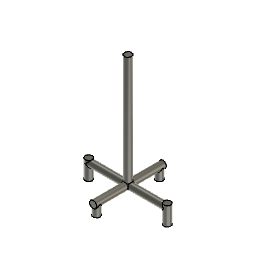
Quad-Ended Pendulum v1 (Autodesk Fusion 360 design; units mm, degrees)
Autodesk Fusion 360 part; units mm, degrees
sketch "Sketch1" plane through (0, 0, 0) normal (0, 0, 1) x (1, 0, 0)
  circle A0 centre (-42, 0) radius 8
  circle A1 centre (138, 0) radius 8
  dimension "d1" = 16
  dimension "d2" = 16
  dimension "d3" = 180
  measures "d1" diameter of A0
  measures "d2" diameter of A1
  measures "d3" distance of A0.centre A1.centre
extrude "Extrude1" add sketch "Sketch1" along normal blind 42 makes body 1 at (145.9901, -0.3988, 28) makes body 2 at (-34.0099, -0.3988, 28)
sketch "Sketch2" plane through (0, 0, 0) normal (1, 0, 0) x (0, 1, 0)
  line L0 (8, 42) -> (-8, 42)
  line L1 (8, 42) -> (-8, 42)
  line L2 (8, 0) -> (-8, 0)
  line L3 (0, 42) -> (0, 34)
  circle A0 centre (0, 34) radius 8
  constraint midpoint L0 L3.start
  constraint perpendicular L1 L3
  constraint coincident L3.end A0.centre
  constraint coincident L3.start A0
extrude "Extrude2" add sketch "Sketch2" along normal up to surface end surface at (-42.1444, 7.9987, 28) on bodies 2 bodies 2
extrude "Extrude3" add 1 faces at (0, 1.5148, 36.1946) along direction (1, 0, 0) up to surface end surface at (134.5104, -7.1988, 28) on bodies 1 2 bodies 2 1
ref_plane "WorkPlane1" through (49.9306, 0, 42) normal (0, 0, 1) x (0, -1, 0)
sketch "Sketch3" plane through (49.9306, 0, 42) normal (0, 0, 1) x (1, 0, 0)
  circle A0 centre (-91.9306, 0) radius 8
  ellipse E0 centre (88.0694, 0) end of major axis (96.0694, 0) minor radius 8 (88.0694, 8) -> (88.0694, -8) ccw
  ellipse E1 centre (88.0694, 0) end of major axis (80.0694, 0) minor radius 8 (80.0694, 0) -> (88.0694, -8) ccw
  ellipse E2 centre (88.0694, 0) end of major axis (80.0694, 0) minor radius 8 (88.0694, 8) -> (80.0694, 0) ccw
  ellipse E3 centre (-91.9306, 0) end of major axis (-83.9306, 0) minor radius 8 (-91.9306, -8) -> (-91.9306, 8) ccw
  ellipse E4 centre (-91.9306, 0) end of major axis (-99.9306, 0) minor radius 8 (-83.9306, 0) -> (-91.9306, 8) ccw
  ellipse E5 centre (-91.9306, 0) end of major axis (-99.9306, 0) minor radius 8 (-91.9306, -8) -> (-83.9306, 0) ccw
  circle A1 centre (88.0694, 0) radius 8
  line L0 (-91.9306, 0) -> (88.0694, 0) construction
  circle A2 centre (-1.9306, 0) radius 8
  dimension "d11" = 16
  constraint coincident A0.centre E3.centre
  constraint coincident E0.centre E1.centre
  constraint midpoint L0 A2.centre
  measures "d11" diameter of A2
extrude "Extrude4" add sketch "Sketch3" against normal blind 8 contours A2 bodies 2
extrude "Extrude5" add 1 faces at (51.2076, -2.1946, 42) along direction (0, 0, 1) blind 250 on bodies 2 bodies 2
ref_plane "WorkPlane2" through (10.2995, -8, 34) normal (0, -1, 0) x (0, 0, -1)
ref_plane "WorkPlane3" through (36.4804, 8, 34) normal (0, 1, 0) x (0, 0, 1)
ref_plane "WorkPlane4" through (36.4804, 0, 34) normal (0, 1, 0) x (0, 0, 1)
sketch "Sketch4" plane through (36.4804, 0, 34) normal (0, 1, 0) x (1, 0, 0)
  line L0 (19.5196, -8) -> (11.5196, 0)
  line L1 (11.5196, 0) -> (3.5196, -8)
  line L2 (101.5196, 0) -> (93.5196, 8)
  line L3 (93.5196, -8) -> (101.5196, 0)
  line L4 (93.5196, -8) -> (101.5196, 0)
  line L5 (-70.4804, 8) -> (-78.4804, 0)
  line L6 (-78.4804, 0) -> (-70.4804, -8)
  line L7 (-78.4804, 0) -> (-70.4804, -8)
  circle A0 centre (11.5196, 0) radius 8
  point P0 (11.5196, 0)
  dimension "d18" = 16
  constraint coincident P0 L0.end
  measures "d18" diameter of A0
extrude "Extrude6" add sketch "Sketch4" along normal mid plane 160 bodies 2
ref_plane "WorkPlane5" through (48, -47.7139, 42) normal (0, 0, 1) x (-1, 0, 0)
ref_plane "WorkPlane6" through (48, -50.1111, 26) normal (0, 0, -1) x (1, 0, 0)
ref_plane "WorkPlane7" through (48, -47.7139, 34) normal (0, 0, 1) x (-1, 0, 0)
sketch "Sketch5" plane through (48, -47.7139, 34) normal (0, 0, 1) x (1, 0, 0)
  line L0 (8, 127.7139) -> (-8, 127.7139)
  arc A0 (5.6569, 53.3707) -> (-5.6569, 53.3707) centre (0, 47.7139) ccw
  line L1 (0, 47.7139) -> (8, 55.7139)
  line L2 (-8, 55.7139) -> (0, 47.7139)
  line L3 (8, 39.7139) -> (0, 47.7139)
  arc A1 (-5.6569, 42.057) -> (5.6569, 42.057) centre (0, 47.7139) ccw
  line L4 (0, 47.7139) -> (-8, 39.7139)
  line L5 (-8, -32.2861) -> (8, -32.2861)
  line L6 (0, -32.2861) -> (0, -24.2861) construction
  line L7 (0, 127.7139) -> (0, 119.7139) construction
  circle A2 centre (0, 119.7139) radius 8
  circle A3 centre (0, -24.2861) radius 8
  dimension "d23" = 8
  dimension "d24" = 8
  dimension "d25" = 16
  constraint midpoint L5 L6.start
  constraint perpendicular L5 L6
  constraint midpoint L0 L7.start
  constraint perpendicular L0 L7
  constraint coincident L7.end A2.centre
  constraint coincident L6.end A3.centre
  constraint coincident L6.start A3
  measures "d23" distance of L6.start L6.end
  measures "d24" distance of L7.start L7.end
  measures "d25" diameter of A2
extrude "Extrude7" add sketch "Sketch5" against normal blind 30 contours A2 | A3 bodies 2
extrude "Extrude8" cut 2 faces at (51.8167, -69.0697, 4) (51.3768, 73.3253, 4) along direction (0, 0, 1) blind 5 on bodies 2 bodies 2
